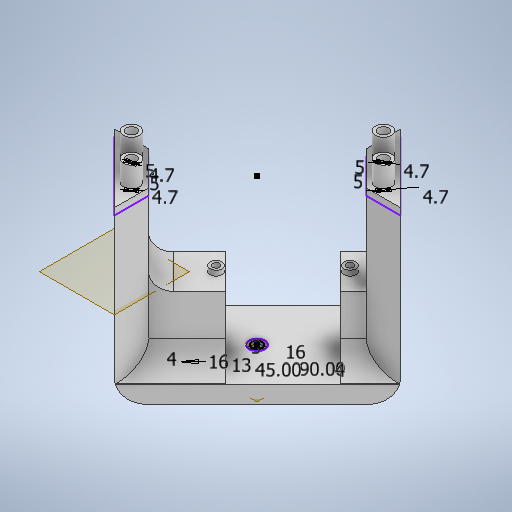
# Autodesk Inventor part: Overhead_Bracket
Saved by Autodesk Inventor 2025.1 (Build 291241000, 241)
## iProperties
Created: 2025-01-24
Part Number: Overhead_Bracket
Material: Generic
Document SubType Name: Modeling
Designer: m_kni
Density: 1 g/cm^3
Appearance: Default
Author: m_kni
## iProperties of the stored document Overhead_Bracket_3DPrint.ipt
Created: 2025-01-30
Part Number: Overhead_Bracket_3DPrint
Material: Generic
Document SubType Name: Modeling
Designer: m_kni
Density: 1 g/cm^3
Appearance: Default
Author: m_kni
Autodesk Inventor part; units mm, degrees
ref_plane "YZ Plane" through (0, 0, 0) normal (1, 0, 0) x (0, 1, 0)
ref_plane "XZ Plane" through (0, 0, 0) normal (0, 1, 0) x (-1, 0, 0)
ref_plane "XY Plane" through (0, 0, 0) normal (0, 0, 1) x (1, 0, 0)
sketch "Sketch1" plane through (0, 0, 0) normal (0, 1, 0) x (-1, 0, 0)
  line L0 (-31.1582, -10.9525) -> (-11.1582, -30.9525)
  line L1 (-11.1582, -20.9525) -> (-21.1582, -10.9525)
  line L2 (10.8418, 21.0475) -> (20.8418, 11.0475)
  line L3 (30.8418, 11.0475) -> (10.8418, 31.0475)
  line L4 (-11.1582, -30.9525) -> (-11.1582, -20.9525)
  line L5 (-21.1582, -10.9525) -> (-31.1582, -10.9525)
  line L6 (10.8418, 21.0475) -> (10.8418, 31.0475)
  line L7 (20.8418, 11.0475) -> (30.8418, 11.0475)
  line L8 (25.8418, 11.0475) -> (10.8418, 26.0475)
  line L9 (-11.1582, -25.9525) -> (-26.1582, -10.9525)
  line L10 (-16.1582, -15.9525) -> (-21.1582, -20.9525)
  line L11 (15.8418, 16.0475) -> (20.8418, 21.0475)
  circle A0 centre (-15.1227, -21.9881) radius 2.35
  circle A1 centre (-22.1938, -14.917) radius 2.35
  circle A2 centre (21.8773, 15.0119) radius 2.35
  circle A3 centre (14.8062, 22.083) radius 2.35
  point P0 (0, 0)
  point P1 (0, 0)
  dimension "d0" = 4.7
  dimension "d1" = 5
  dimension "d2" = 5
  dimension "d3" = 4.7
  dimension "d4" = 4.7
  dimension "d5" = 4.7
  dimension "d6" = 5
  dimension "d7" = 5
  constraints: 24 end point, 8 midpoint, 4 centre point, 4 point on line, 2 perpendicular, 1 coincident, 1 vertical
  measures "d0" diameter of A0
  measures "d1" distance from line of L10 A0.centre
  measures "d2" distance from line of L10 A1.centre
  measures "d3" diameter of A1
  measures "d4" diameter of A2
  measures "d5" diameter of A3
  measures "d6" distance from line of A3.centre L11
  measures "d7" distance from line of L11 A2.centre
extrude "Extrusion1" add sketch "Sketch1" along normal blind 6 contours A1 L9 | L9 A1 | A0 L9 | L9 A0 | A3 L8 | L8 A3 | A2 L8 | L8 A2
extrude "Extrusion2" add sketch "Sketch1" against normal blind 43
sketch "Sketch2" plane through (0, -43, 0) normal (0, -1, 0) x (1, 0, 0)
  line L0 (-30.8418, 11.0475) -> (-20.8418, 11.0475) projected
  line L1 (11.1582, -20.9525) -> (11.1582, -30.9525) projected
  line L2 (-30.8418, 11.0475) -> (11.1582, -30.9525)
  line L3 (-10.8418, 21.0475) -> (-10.8418, 31.0475) projected
  line L4 (-10.8418, 31.0475) -> (31.1582, -10.9525)
  line L5 (-10.8418, 31.0475) -> (-30.8418, 11.0475)
  line L6 (11.1582, -30.9525) -> (31.1582, -10.9525)
  point P0 (0, 0)
  constraints: 8 end point, 1 parallel
extrude "Extrusion3" add sketch "Sketch2" along normal blind 5
sketch "Sketch3" plane through (0, -48, 0) normal (0, -1, 0) x (1, 0, 0)
  circle A0 centre (0, 0) radius 6.5
  line L0 (0, 0) -> (11.3137, -11.3137)
  line L1 (0, 0) -> (16, 0) construction
  line L2 (11.3137, -11.3137) -> (14.1421, -8.4853)
  line L3 (14.1421, -8.4853) -> (6.0192, -0.3623)
  line L4 (0, 0) -> (-11.3137, 11.3137)
  line L5 (-11.3137, 11.3137) -> (-8.4853, 14.1421)
  line L6 (-8.4853, 14.1421) -> (6.0192, -0.3623)
  line L7 (-11.3137, 11.3137) -> (-14.1421, 8.4853)
  line L8 (-14.1421, 8.4853) -> (8.4853, -14.1421)
  line L9 (8.4853, -14.1421) -> (11.3137, -11.3137)
  point P0 (-6.4513, 0.7944)
  point P1 (0.7944, -6.4513)
  point P2 (6.4513, -0.7944)
  point P3 (-0.7944, 6.4513)
  dimension "d14" = 13
  dimension "d15" = 16
  dimension "d16" = 45
  dimension "d17" = 4
  dimension "d18" = 90
  dimension "d19" = 16
  dimension "d20" = 4
  constraints: 20 end point, 5 perpendicular, 1 centre point, 1 coincident, 1 equal length, 1 horizontal
  measures "d14" diameter of A0
  measures "d15" distance of L0.start L0.end
  measures "d16" angle of L0 L1
  measures "d17" distance of L0.end L2.end
  measures "d18" angle of L3 L2
  measures "d19" distance of L0.start L4.end
  measures "d20" distance of L4.end L7.end
ref_plane "Work Plane3" through (0, -46.5, 0) normal (0, -1, 0) x (1, 0, 0)
sketch "Sketch4" plane through (0, -46.5, 0) normal (0, -1, 0) x (1, 0, 0)
  circle A0 centre (0, 0) radius 2.25
  dimension "d23" = 4.5
  constraints: 1 centre point, 1 coincident
  measures "d23" diameter of A0
extrude "Extrusion5" cut sketch "Sketch4" against normal blind 3
sketch "Sketch5" plane through (-14.8062, 6, 22.083) normal (0, 1, 0) x (1, 0, 0)
  circle A0 centre (0, 0) radius 1.5
  circle A1 centre (-7.0711, 7.0711) radius 2.35 projected
  circle A2 centre (-7.0711, 7.0711) radius 1.5
  circle A3 centre (37, 37) radius 2.35 projected
  circle A4 centre (29.9289, 44.0711) radius 2.35 projected
  circle A5 centre (37, 37) radius 2.35 projected
  circle A6 centre (37, 37) radius 1.5
  circle A7 centre (29.9289, 44.0711) radius 1.5
  point P0 (14.8062, 22.083)
  dimension "d26" = 3
  dimension "d27" = 3
  dimension "d28" = 3
  dimension "d29" = 3
  constraints: 4 centre point, 3 coincident
  measures "d26" diameter of A0
  measures "d27" diameter of A2
  measures "d28" diameter of A6
  measures "d29" diameter of A7
extrude "Extrusion6" cut sketch "Sketch5" against normal blind 8 contours A0 | A2 | A6 | A7
sketch "Sketch6" plane through (0, 0, 0) normal (0, 1, 0) x (1, 0, 0)
  circle A0 centre (15.1227, 21.9881) radius 2.35 projected
  circle A1 centre (15.1227, 21.9881) radius 1.5 projected
  circle A2 centre (22.1938, 14.917) radius 2.35 projected
  circle A3 centre (22.1938, 14.917) radius 1.5 projected
  circle A4 centre (-21.8773, -15.0119) radius 2.35 projected
  circle A5 centre (-21.8773, -15.0119) radius 1.5 projected
  circle A6 centre (-14.8062, -22.083) radius 2.35 projected
  circle A7 centre (-14.8062, -22.083) radius 1.5 projected
  point P0 (0, 0)
ref_plane "Work Plane1" through (0, -24.275, 0) normal (0, 1, 0) x (1, 0, 0)
sketch "Sketch7" plane through (0, -24.275, 0) normal (0, 1, 0) x (1, 0, 0)
  circle A0 centre (0, 0) radius 2.25 projected
  circle A1 centre (0, 0) radius 2.4
  line L0 (-25.8418, -11.0475) -> (-10.8418, -26.0475) projected
  line L1 (0, 0) -> (-6.0104, -6.0104)
  line L2 (0, 0) -> (13.6472, 13.6472)
  line L3 (0, 0) -> (19.3, 0) construction
  circle A2 centre (-6.0104, -6.0104) radius 1.3
  circle A3 centre (13.6472, 13.6472) radius 1.3
  line L4 (0, 0) -> (-4.5962, -4.5962)
  line L5 (0, 0) -> (6.5, 0) construction
  line L6 (0, 0) -> (0, 9.3002)
  line L7 (0, 0) -> (12.2329, 12.2329)
  line L8 (-10.8418, -21.0475) -> (-20.8418, -11.0475) projected
  line L9 (11.1582, 20.9525) -> (21.1582, 10.9525) projected
  line L10 (-10.8418, -21.0475) -> (0.5066, -9.699)
  line L11 (0.5066, -9.699) -> (-4.5962, -4.5962)
  line L12 (-30.8418, -11.0475) -> (-20.8418, -11.0475) projected
  line L13 (-20.8418, -11.0475) -> (-9.4934, 0.301)
  line L14 (-9.4934, 0.301) -> (-4.5962, -4.5962)
  line L15 (21.1582, 10.9525) -> (11.1582, 20.9525)
  line L16 (12.2329, 12.2329) -> (7.3358, 17.1301)
  line L17 (7.3358, 17.1301) -> (11.1582, 20.9525)
  line L18 (12.2329, 12.2329) -> (17.3358, 7.1301)
  line L19 (17.3358, 7.1301) -> (21.1582, 10.9525)
  circle A4 centre (13.6472, 13.6472) radius 1
  circle A5 centre (-6.0104, -6.0104) radius 1
  dimension "d36" = 4.8
  dimension "d37" = 8.5
  dimension "d38" = 19.3
  dimension "d39" = 45
  dimension "d40" = 2.6
  dimension "d41" = 2.6
  dimension "d42" = 6.5
  dimension "d43" = 135
  dimension "d44" = 135
  dimension "d45" = 17.3
  dimension "d51" = 2
  dimension "d52" = 2
  constraints: 32 end point, 7 point on line, 5 centre point, 5 coincident, 5 perpendicular, 2 equal length, 2 horizontal, 1 collinear, 1 parallel
  measures "d36" diameter of A1
  measures "d37" distance of L1.start L1.end
  measures "d38" distance of L1.start L2.end
  measures "d39" angle of L3 L2
  measures "d40" diameter of A2
  measures "d41" diameter of A3
  measures "d42" distance of L1.start L4.end
  measures "d43" angle of L4 L5
  measures "d44" angle of L1 L6
  measures "d45" distance of L1.start L7.end
  measures "d51" diameter of A4
  measures "d52" diameter of A5
extrude "Extrusion7" add sketch "Sketch7" against normal up to surface (18.725 mm away) contours A2 | A3 | L8 L13 L14 L11 L10 | L9 L19 L18 L16 L17
fillet "Fillet6" radius 6.7625 2 edges at (21.1582, -48, -20.9525) (-20.8418, -48, 21.0475)
sketch "Sketch8" plane through (0, -43, 0) normal (0, 1, 0) x (1, 0, 0)
  circle A0 centre (0, 0) radius 2.25 projected
  circle A1 centre (0, 0) radius 2.25
  circle A2 centre (0, 0) radius 1.5
  dimension "d53" = 3
  constraints: 2 centre point, 2 coincident
  measures "d53" diameter of A2
extrude "Extrusion8" cut sketch "Sketch8" against normal blind 4.85 contours A2
extrude "Extrusion9" cut sketch "Sketch8" against normal blind 1.5 contours A0 | A2
fillet "Fillet7" radius 6.7625 4 edges at (-15.1676, -43, 5.3733) (9.247, -43, -19.0413) (19.247, -43, -9.0413) (-5.1676, -43, 15.3733)
ref_plane "Work Plane2" through (0, -46.5, 0) normal (0, -1, 0) x (1, 0, 0)
sketch "Sketch9" plane through (0, -46.5, 0) normal (0, -1, 0) x (1, 0, 0)
  circle A0 centre (0, 0) radius 2.25
  circle A1 centre (0, 0) radius 1.5
  dimension "d59" = 3
  constraints: 2 centre point, 2 coincident
  measures "d59" diameter of A1
extrude "Extrusion10" add sketch "Sketch9" against normal blind 2
fillet "Fillet8" radius 5.175 1 edges at (-15.8418, -24.275, 16.0475)
extrude "Extrusion11" add sketch "Sketch1" along normal blind 2 contours L5 L9 A1 L10 L0 | L10 L9 A0 L4 L0 | L5 L1 L10 L9 A1 | L10 L1 L4 L9 A0 | L6 L8 A3 L11 L2 | L11 L8 A2 L7 L2 | L6 L3 L11 L8 A3 | L11 L3 L7 L8 A2
sketch "Sketch10" plane through (-14.8062, 6, 22.083) normal (0, 1, 0) x (1, 0, 0)
  circle A0 centre (0, 0) radius 1.5 projected
  circle A1 centre (0, 0) radius 2.35 projected
  circle A2 centre (-7.0711, 7.0711) radius 2.35 projected
  circle A3 centre (-7.0711, 7.0711) radius 1.5 projected
  circle A4 centre (37, 37) radius 2.35 projected
  circle A5 centre (37, 37) radius 1.5 projected
  circle A6 centre (29.9289, 44.0711) radius 1.5 projected
  circle A7 centre (29.9289, 44.0711) radius 2.35 projected
  point P0 (14.8062, 22.083)
extrude "Extrusion12" add sketch "Sketch10" along normal blind 2
sketch "Sketch11" plane through (0, -48, 0) normal (0, -1, 0) x (1, 0, 0)
  circle A0 centre (0, 17.1) radius 0.85
  circle A1 centre (0, -17.1) radius 0.85
  line L0 (0, 0) -> (0, 17.1) construction
  line L1 (0, -17.1) -> (0, 0) construction
  circle A2 centre (0, 17.1) radius 2.65
  circle A3 centre (0, -17.1) radius 2.65
  circle A4 centre (0, 0) radius 6
  line L2 (-2.627, -17.4484) -> (-4.4, -4.0792)
  line L3 (4.4, -4.0792) -> (2.627, -17.4484)
  line L4 (-4.4, 4.0792) -> (-2.627, 17.4484)
  line L5 (2.627, 17.4484) -> (4.4, 4.0792)
  circle A5 centre (0, 0) radius 1.5
  circle A6 centre (0, 0) radius 4
  circle A7 centre (-12.0915, 12.0915) radius 2.65
  line L6 (-10.4803, 14.1954) -> (0.2268, 5.9957)
  line L7 (-5.9957, -0.2268) -> (-14.1954, 10.4803)
  circle A8 centre (0, 0) radius 6
  line L8 (10.4803, -14.1954) -> (-0.2268, -5.9957)
  circle A9 centre (12.0915, -12.0915) radius 2.65
  line L9 (5.9957, 0.2268) -> (14.1954, -10.4803)
  circle A10 centre (0, 0) radius 4
  circle A11 centre (0, 0) radius 1.5
  dimension "d67" = 1.7
  dimension "d68" = 1.7
  dimension "d69" = 17.1
  dimension "d70" = 5.3
  dimension "d71" = 5.3
  dimension "d72" = 12
  dimension "d73" = 8.8
  dimension "d74" = 8.8
  dimension "d75" = 3
  dimension "d76" = 8
  dimension "d79" = 45
  constraints: 20 end point, 16 point on circle, 12 centre point, 8 coincident, 4 tangent, 3 equal length, 1 collinear, 1 vertical, 23 other
  measures "d67" diameter of A1
  measures "d68" diameter of A0
  measures "d69" distance of L0.start L0.end
  measures "d70" diameter of A2
  measures "d71" diameter of A3
  measures "d72" diameter of A4
  measures "d73" distance of L5.end L4.start
  measures "d74" distance of L3.start L2.end
  measures "d75" diameter of A5
  measures "d76" diameter of A6
extrude "Extrusion13" cut sketch "Sketch11" against normal blind 3 contours A4 | L6 A4 L4 | L4 A4 L7 A7 L6 | L9 A9 L8 L3 A4 | A7 | A9 | L3 L8 A4 | A5 | A6
sketch "Sketch12" plane through (0, 2, 0) normal (0, 1, 0) x (1, 0, 0)
  line L0 (-10.8418, -31.0475) -> (-30.8418, -11.0475) projected
  line L1 (-10.8418, -31.0475) -> (-30.8418, -11.0475)
  line L2 (-20.8418, -21.0475) -> (21.1582, 20.9525)
  line L3 (11.1582, 30.9525) -> (31.1582, 10.9525) projected
  line L4 (-20.8418, -11.0475) -> (-30.4054, -11.0475) projected
  line L5 (-7.1825, -17.3882) -> (-10.8418, -21.0475) projected
  line L6 (-20.8418, -11.0475) -> (-10.8418, -21.0475)
  line L7 (11.1582, 20.9525) -> (21.1582, 10.9525) projected
  line L8 (11.1582, 20.9525) -> (21.1582, 10.9525)
  circle A0 centre (22.1938, 14.917) radius 1.5 projected
  line L9 (21.1582, 10.9525) -> (31.1582, 10.9525) projected
  line L10 (31.1582, 10.9525) -> (11.1582, 30.9525) projected
  line L11 (11.1582, 30.9525) -> (11.1582, 20.9525) projected
  line L12 (11.1582, 20.9525) -> (21.1582, 10.9525) projected
  circle A1 centre (22.1938, 14.917) radius 2.35 projected
  circle A2 centre (15.1227, 21.9881) radius 2.35 projected
  circle A3 centre (15.1227, 21.9881) radius 1.5 projected
  line L13 (22.1938, 14.917) -> (15.1227, 21.9881)
  circle A4 centre (18.6582, 18.4525) radius 0.7254
  circle A5 centre (-14.8062, -22.083) radius 1.5 projected
  circle A6 centre (-21.8773, -15.0119) radius 1.5 projected
  line L14 (-14.8062, -22.083) -> (-21.8773, -15.0119)
  circle A7 centre (-18.3418, -18.5475) radius 1
  point P0 (0, 0)
  dimension "d83" = 2
  constraints: 12 end point, 4 midpoint, 2 centre point, 2 collinear, 1 perpendicular
  measures "d83" diameter of A7
extrude "Extrusion14" cut sketch "Sketch12" against normal blind 10 contours A7 L14 L2 | L2 L14 A7 | L14 A7 L2 | L2 A7 L14 | A4 L13 L2 | L2 L13 A4 | L13 A4 L2 | L2 A4 L13
sketch "Sketch13" plane through (0, -24.275, 0) normal (0, 1, 0) x (1, 0, 0)
  circle A0 centre (-6.0104, -6.0104) radius 1 projected
  circle A1 centre (13.6472, 13.6472) radius 1 projected
  circle A2 centre (-6.0104, -6.0104) radius 1
  circle A3 centre (13.6472, 13.6472) radius 1
  circle A4 centre (13.6472, 13.6472) radius 1.75
  circle A5 centre (-6.0104, -6.0104) radius 1.75
  point P0 (0, 0)
  dimension "d86" = 3.5
  dimension "d87" = 3.5
  constraints: 4 centre point, 4 coincident, 2 concentric
  measures "d86" diameter of A4
  measures "d87" diameter of A5
extrude "Extrusion15" add sketch "Sketch13" along normal blind 1.5
equation "\"d71\" = d70"
equation "\"d74\" = d73"
body "Solid1"
